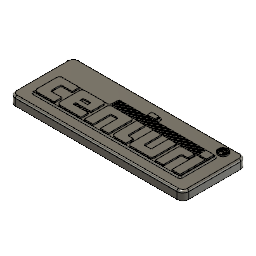
Centuri (Autodesk Fusion 360 design; units mm, degrees)
Autodesk Fusion 360 part; units mm, degrees
note: some values were not read from the file. Set by a fixed rule: which sketch regions a step uses.
sketch "Sketch1" plane through (0, 0, 0) normal (0, 1, 0) x (1, 0, 0)
  line L0 (168.1224, -0.1324) -> (6.1323, -0.1324)
  line L1 (0.1323, -6.1324) -> (0.1323, -58.135)
  line L2 (6.1323, -64.135) -> (168.1224, -64.135)
  line L3 (174.1224, -58.135) -> (174.1224, -6.1324)
  arc A0 (6.1323, -0.1324) -> (0.1323, -6.1324) centre (6.1323, -6.1324) ccw
  arc A1 (0.1323, -58.135) -> (6.1323, -64.135) centre (6.1323, -58.135) ccw
  arc A2 (174.1224, -6.1324) -> (168.1224, -0.1324) centre (168.1224, -6.1324) ccw
  arc A3 (168.1224, -64.135) -> (174.1224, -58.135) centre (168.1224, -58.135) ccw
  dimension "d26" = 6
  dimension "d27" = 6
  dimension "d28" = 6
  dimension "d29" = 6
  measures "d26" radius of A0
  measures "d27" radius of A1
  measures "d28" radius of A2
  measures "d29" radius of A3
extrude "Extrude1" add sketch "Sketch1" along normal blind 8.7
sketch "Sketch2" plane through (0, 8.7, 0) normal (0, 1, 0) x (-1, 0, 0)
  line L0 (-174.1224, 58.135) -> (-174.1224, 6.1324)
  line L1 (-168.1224, 0.1324) -> (-6.1323, 0.1324)
  line L2 (-0.1323, 6.1324) -> (-0.1323, 58.135)
  line L3 (-6.1323, 64.135) -> (-168.1224, 64.135)
  line L4 (-174.1224, 6.1324) -> (-174.1224, 58.135)
  line L5 (-168.1224, 64.135) -> (-6.1323, 64.135)
  line L6 (-0.1323, 58.135) -> (-0.1323, 6.1324)
  line L7 (-6.1323, 0.1324) -> (-168.1224, 0.1324)
  arc A0 (-168.1224, 64.135) -> (-174.1224, 58.135) centre (-168.1224, 58.135) ccw
  arc A1 (-174.1224, 6.1324) -> (-168.1224, 0.1324) centre (-168.1224, 6.1324) ccw
  arc A2 (-6.1323, 0.1324) -> (-0.1323, 6.1324) centre (-6.1323, 6.1324) ccw
  arc A3 (-0.1323, 58.135) -> (-6.1323, 64.135) centre (-6.1323, 58.135) ccw
  arc A4 (-168.1224, 64.135) -> (-174.1224, 58.135) centre (-168.1224, 58.135) ccw
  arc A5 (-0.1323, 58.135) -> (-6.1323, 64.135) centre (-6.1323, 58.135) ccw
  arc A6 (-6.1323, 0.1324) -> (-0.1323, 6.1324) centre (-6.1323, 6.1324) ccw
  arc A7 (-174.1224, 6.1324) -> (-168.1224, 0.1324) centre (-168.1224, 6.1324) ccw
  line L8 (-61.1568, 23.5465) -> (-61.1568, 18.1721)
  line L9 (-13.3787, 24.5465) -> (-60.1568, 24.5465)
  line L10 (-160.8508, 51.6795) -> (-160.8508, 18.1721)
  line L11 (-158.8508, 16.1721) -> (-101.0747, 16.1721)
  line L12 (-100.0747, 12.3992) -> (-100.0747, 15.1721)
  line L13 (-91.1387, 10.3992) -> (-98.0747, 10.3992)
  line L14 (-89.1387, 12.3992) -> (-89.1387, 15.1721)
  line L15 (-88.1387, 16.1721) -> (-63.1568, 16.1721)
  line L16 (-13.3787, 53.6795) -> (-158.8508, 53.6795)
  line L17 (-11.3787, 51.6795) -> (-11.3787, 26.5465)
  arc A8 (-63.1568, 16.1721) -> (-61.1568, 18.1721) centre (-63.1568, 18.1721) ccw
  arc A9 (-91.1387, 10.3992) -> (-89.1387, 12.3992) centre (-91.1387, 12.3992) ccw
  arc A10 (-100.0747, 12.3992) -> (-98.0747, 10.3992) centre (-98.0747, 12.3992) ccw
  arc A11 (-160.8508, 18.1721) -> (-158.8508, 16.1721) centre (-158.8508, 18.1721) ccw
  arc A12 (-158.8508, 53.6795) -> (-160.8508, 51.6795) centre (-158.8508, 51.6795) ccw
  arc A13 (-11.3787, 51.6795) -> (-13.3787, 53.6795) centre (-13.3787, 51.6795) ccw
  arc A14 (-13.3787, 24.5465) -> (-11.3787, 26.5465) centre (-13.3787, 26.5465) ccw
  arc A15 (-60.1568, 24.5465) -> (-61.1568, 23.5465) centre (-60.1568, 23.5465) ccw
  arc A16 (-88.1387, 16.1721) -> (-89.1387, 15.1721) centre (-88.1387, 15.1721) ccw
  arc A17 (-100.0747, 15.1721) -> (-101.0747, 16.1721) centre (-101.0747, 15.1721) ccw
  dimension "d32" = 2
  dimension "d33" = 2
  dimension "d34" = 2
  dimension "d35" = 2
  dimension "d36" = 2
  dimension "d37" = 2
  dimension "d38" = 2
  dimension "d39" = 1
  dimension "d40" = 1
  dimension "d41" = 1
  measures "d32" radius of A8
  measures "d33" radius of A9
  measures "d34" radius of A10
  measures "d35" radius of A11
  measures "d36" radius of A12
  measures "d37" radius of A13
  measures "d38" radius of A14
  measures "d39" radius of A15
  measures "d40" radius of A16
  measures "d41" radius of A17
extrude "Extrude2" add sketch "Sketch2" along normal blind 1.2 contours L8 L9 L10 L11 L12 L13 L14 L15 L16 L17 A8 A9 A10 A11 A12 A13 A14 A15 A16 A17
sketch "Sketch3" plane through (0, 9.9, 0) normal (0, 1, 0) x (-1, 0, 0)
  spline S0 degree 2 poles (-32.9928, 26.8178) (-19.083, 26.7952) (-15.8247, 26.8178) knots 0 0 0 1 1 1
  spline S1 degree 3 poles (-15.8247, 26.8178) (-14.6011, 26.8261) (-13.0709, 27.9977) (-13.0639, 29.2054) knots 0 0 0 0 1 1 1 1
  spline S2 degree 3 poles (-13.0639, 29.2054) (-13.0417, 32.9886) (-13.0526, 45.265) (-13.0639, 49.042) knots 0 0 0 0 1 1 1 1
  spline S3 degree 3 poles (-13.0639, 49.042) (-13.0677, 50.37) (-14.4791, 51.9469) (-15.8247, 51.9487) knots 0 0 0 0 1 1 1 1
  spline S4 degree 2 poles (-15.8247, 51.9487) (-19.0795, 51.9532) (-32.9674, 51.9487) knots 0 0 0 1 1 1
  line L0 (-32.9674, 51.9487) -> (-32.9928, 44.3788)
  spline S5 degree 2 poles (-32.9928, 44.3788) (-24.5516, 44.3725) (-22.6517, 44.3788) knots 0 0 0 1 1 1
  spline S6 degree 3 poles (-22.6517, 44.3788) (-22.0091, 44.3809) (-21.5788, 43.4319) (-21.5873, 42.7928) knots 0 0 0 0 1 1 1 1
  spline S7 degree 3 poles (-21.5873, 42.7928) (-21.6066, 41.3105) (-21.5967, 36.9365) (-21.5873, 35.4147) knots 0 0 0 0 1 1 1 1
  spline S8 degree 3 poles (-21.5873, 35.4147) (-21.5834, 34.8089) (-22.0316, 33.8745) (-22.6453, 33.8752) knots 0 0 0 0 1 1 1 1
  spline S9 degree 2 poles (-22.6453, 33.8752) (-24.5882, 33.8783) (-32.9928, 33.8752) knots 0 0 0 1 1 1
  line L1 (-32.9928, 33.8752) -> (-32.9928, 26.8178)
  spline S10 degree 3 poles (-56.7768, 26.8178) (-53.3593, 26.806) (-42.7162, 26.8025) (-39.2193, 26.8178) knots 0 0 0 0 1 1 1 1
  spline S11 degree 3 poles (-39.2193, 26.8178) (-37.8445, 26.8237) (-35.8622, 27.8316) (-35.8661, 29.1884) knots 0 0 0 0 1 1 1 1
  spline S12 degree 3 poles (-35.8661, 29.1884) (-35.8777, 33.0541) (-35.8672, 45.7175) (-35.8661, 49.4432) knots 0 0 0 0 1 1 1 1
  spline S13 degree 3 poles (-35.8661, 49.4432) (-35.8658, 50.8266) (-37.8171, 51.9476) (-39.2193, 51.9487) knots 0 0 0 0 1 1 1 1
  spline S14 degree 2 poles (-39.2193, 51.9487) (-43.0994, 51.9508) (-59.7334, 51.9487) knots 0 0 0 1 1 1
  line L2 (-59.7334, 51.9487) -> (-59.7334, 44.3788)
  spline S15 degree 2 poles (-59.7334, 44.3788) (-47.3321, 44.3802) (-44.8507, 44.3788) knots 0 0 0 1 1 1
  spline S16 degree 3 poles (-44.8507, 44.3788) (-44.0281, 44.3781) (-44.0281, 41.943) (-44.8507, 41.944) knots 0 0 0 0 1 1 1 1
  spline S17 degree 2 poles (-44.8507, 41.944) (-47.3567, 41.9471) (-59.7334, 41.944) knots 0 0 0 1 1 1
  spline S18 degree 2 poles (-59.7334, 41.944) (-59.732, 31.8277) (-59.7334, 29.1884) knots 0 0 0 1 1 1
  spline S19 degree 3 poles (-59.7334, 29.1884) (-59.7342, 27.9349) (-58.0465, 26.8219) (-56.7768, 26.8178) knots 0 0 0 0 1 1 1 1
  line L3 (-44.6029, 37.6033) -> (-52.1177, 37.6033)
  spline S20 degree 2 poles (-52.1177, 37.6033) (-52.1195, 35.5658) (-52.1177, 35.0104) knots 0 0 0 1 1 1
  spline S21 degree 3 poles (-52.1177, 35.0104) (-52.117, 34.6915) (-51.7641, 34.3481) (-51.4621, 34.3488) knots 0 0 0 0 1 1 1 1
  spline S22 degree 3 poles (-51.4621, 34.3488) (-50.3271, 34.3526) (-46.4378, 34.3473) (-45.2915, 34.3488) knots 0 0 0 0 1 1 1 1
  spline S23 degree 3 poles (-45.2915, 34.3488) (-44.9814, 34.3496) (-44.6039, 34.683) (-44.6029, 35.0104) knots 0 0 0 0 1 1 1 1
  spline S24 degree 2 poles (-44.6029, 35.0104) (-44.6011, 35.5814) (-44.6029, 37.6033) knots 0 0 0 1 1 1
  line L4 (-63.1696, 51.9483) -> (-71.8638, 51.9483)
  spline S25 degree 2 poles (-71.8638, 51.9483) (-71.8656, 38.5103) (-71.8638, 35.6595) knots 0 0 0 1 1 1
  spline S26 degree 3 poles (-71.8638, 35.6595) (-71.8634, 34.7649) (-71.8395, 34.1505) (-72.4016, 34.1501) knots 0 0 0 0 1 1 1 1
  spline S27 degree 3 poles (-72.4016, 34.1501) (-73.5093, 34.1491) (-77.3834, 34.1456) (-78.5466, 34.1501) knots 0 0 0 0 1 1 1 1
  spline S28 degree 3 poles (-78.5466, 34.1501) (-79.1909, 34.1526) (-79.1888, 34.8162) (-79.1895, 35.6595) knots 0 0 0 0 1 1 1 1
  spline S29 degree 2 poles (-79.1895, 35.6595) (-79.1923, 38.6438) (-79.1895, 51.9071) knots 0 0 0 1 1 1
  line L5 (-79.1895, 51.9071) -> (-87.5653, 51.9483)
  spline S30 degree 2 poles (-87.5653, 51.9483) (-87.5688, 33.4546) (-87.5653, 29.1884) knots 0 0 0 1 1 1
  spline S31 degree 3 poles (-87.5653, 29.1884) (-87.5646, 28.1107) (-86.4298, 26.8171) (-85.3377, 26.8178) knots 0 0 0 0 1 1 1 1
  spline S32 degree 3 poles (-85.3377, 26.8178) (-81.607, 26.8202) (-69.4534, 26.8101) (-65.7431, 26.8178) knots 0 0 0 0 1 1 1 1
  spline S33 degree 3 poles (-65.7431, 26.8178) (-64.5697, 26.8202) (-63.1696, 28.0306) (-63.1696, 29.1884) knots 0 0 0 0 1 1 1 1
  spline S34 degree 2 poles (-63.1696, 29.1884) (-63.1689, 33.4147) (-63.1696, 51.9483) knots 0 0 0 1 1 1
  line L6 (-90.6576, 26.8178) -> (-98.9156, 26.8178)
  spline S35 degree 2 poles (-98.9156, 26.8178) (-98.9159, 40.6126) (-98.9156, 43.5182) knots 0 0 0 1 1 1
  spline S36 degree 3 poles (-98.9156, 43.5182) (-98.9152, 43.9294) (-99.3947, 44.3788) (-99.8116, 44.3788) knots 0 0 0 0 1 1 1 1
  spline S37 degree 2 poles (-99.8116, 44.3788) (-99.8559, 44.3788) (-104.8904, 44.3788) knots 0 0 0 1 1 1
  line L7 (-104.8904, 44.3788) -> (-104.946, 51.9532)
  spline S38 degree 2 poles (-104.946, 51.9532) (-96.959, 51.9452) (-94.523, 51.9532) knots 0 0 0 1 1 1
  spline S39 degree 3 poles (-94.523, 51.9532) (-90.2713, 51.9667) (-90.6439, 48.9779) (-90.6435, 47.4106) knots 0 0 0 0 1 1 1 1
  spline S40 degree 2 poles (-90.6435, 47.4106) (-90.6425, 43.2176) (-90.6576, 26.8178) knots 0 0 0 1 1 1
  line L8 (-107.072, 26.8178) -> (-115.2878, 26.8178)
  spline S41 degree 2 poles (-115.2878, 26.8178) (-115.2881, 40.5276) (-115.2878, 43.4547) knots 0 0 0 1 1 1
  spline S42 degree 3 poles (-115.2878, 43.4547) (-115.2878, 43.8323) (-115.5693, 44.3784) (-115.9521, 44.3788) knots 0 0 0 0 1 1 1 1
  spline S43 degree 3 poles (-115.9521, 44.3788) (-117.0559, 44.3791) (-120.8583, 44.3788) (-121.979, 44.3788) knots 0 0 0 0 1 1 1 1
  spline S44 degree 3 poles (-121.979, 44.3788) (-122.3375, 44.3788) (-122.508, 43.8084) (-122.5084, 43.4547) knots 0 0 0 0 1 1 1 1
  spline S45 degree 2 poles (-122.5084, 43.4547) (-122.5105, 40.5287) (-122.5084, 26.8178) knots 0 0 0 1 1 1
  line L9 (-122.5084, 26.8178) -> (-130.83, 26.8178)
  spline S46 degree 2 poles (-130.83, 26.8178) (-130.8286, 44.9394) (-130.83, 49.1325) knots 0 0 0 1 1 1
  spline S47 degree 3 poles (-130.83, 49.1325) (-130.8303, 50.3291) (-129.8661, 51.9483) (-128.543, 51.9494) knots 0 0 0 0 1 1 1 1
  spline S48 degree 3 poles (-128.543, 51.9494) (-124.6333, 51.9528) (-112.8693, 51.9521) (-109.3164, 51.9494) knots 0 0 0 0 1 1 1 1
  spline S49 degree 3 poles (-109.3164, 51.9494) (-108.0865, 51.9487) (-107.0706, 50.2577) (-107.072, 49.1328) knots 0 0 0 0 1 1 1 1
  spline S50 degree 2 poles (-107.072, 49.1328) (-107.0765, 44.9318) (-107.072, 26.8178) knots 0 0 0 1 1 1
  line L10 (-148.6286, 26.8178) -> (-148.6286, 33.5954)
  spline S51 degree 2 poles (-148.6286, 33.5954) (-144.7896, 33.5968) (-143.7112, 33.5954) knots 0 0 0 1 1 1
  spline S52 degree 3 poles (-143.7112, 33.5954) (-142.9807, 33.5943) (-142.2763, 34.5093) (-142.2756, 35.2306) knots 0 0 0 0 1 1 1 1
  spline S53 degree 2 poles (-142.2756, 35.2306) (-142.2735, 38.3037) (-142.2756, 51.9521) knots 0 0 0 1 1 1
  line L11 (-142.2756, 51.9521) -> (-134.2615, 51.9521)
  spline S54 degree 2 poles (-134.2615, 51.9521) (-134.2622, 33.6976) (-134.2615, 29.4065) knots 0 0 0 1 1 1
  spline S55 degree 3 poles (-134.2615, 29.4065) (-134.2612, 27.9849) (-136.2557, 26.8198) (-137.6963, 26.8178) knots 0 0 0 0 1 1 1 1
  spline S56 degree 2 poles (-137.6963, 26.8178) (-140.0743, 26.8143) (-148.6286, 26.8178) knots 0 0 0 1 1 1
  line L12 (-150.7694, 26.8178) -> (-159.0611, 26.8178)
  line L13 (-159.0611, 26.8178) -> (-159.0611, 51.949)
  line L14 (-159.0611, 51.949) -> (-150.7694, 51.8679)
  line L15 (-150.7694, 51.8679) -> (-150.7694, 26.8178)
  spline S57 degree 3 poles (-98.4051, 12.6404) (-98.4051, 12.3033) (-98.1313, 12.0297) (-97.7942, 12.0297) knots 0 0 0 0 1 1 1 1
  line L16 (-97.7942, 12.0297) -> (-91.45, 12.0297)
  spline S58 degree 3 poles (-91.45, 12.0297) (-91.113, 12.0297) (-90.8394, 12.3033) (-90.8394, 12.6404) knots 0 0 0 0 1 1 1 1
  line L17 (-90.8394, 12.6404) -> (-90.8394, 15.7818)
  spline S59 degree 3 poles (-90.8394, 15.7818) (-90.8394, 16.1189) (-91.113, 16.3927) (-91.45, 16.3927) knots 0 0 0 0 1 1 1 1
  line L18 (-91.45, 16.3927) -> (-97.7942, 16.3927)
  spline S60 degree 3 poles (-97.7942, 16.3927) (-98.1313, 16.3927) (-98.4051, 16.1189) (-98.4051, 15.7818) knots 0 0 0 0 1 1 1 1
  line L19 (-98.4051, 15.7818) -> (-98.4051, 12.6404)
  spline S61 degree 2 poles (-64.6658, 17.7949) (-80.3905, 17.7962) (-159.0863, 17.7949) knots 0 0 0 1 1 1
  line L20 (-159.0863, 17.7949) -> (-159.0863, 25.3701)
  spline S62 degree 2 poles (-159.0863, 25.3701) (-80.3944, 25.3701) (-64.6658, 25.3701) knots 0 0 0 1 1 1
  spline S63 degree 3 poles (-64.6658, 25.3701) (-64.173, 25.3701) (-64.1386, 24.2219) (-64.6658, 24.2219) knots 0 0 0 0 1 1 1 1
  spline S64 degree 3 poles (-64.6658, 24.2219) (-79.0329, 24.2233) (-136.3969, 24.2233) (-150.7538, 24.2219) knots 0 0 0 0 1 1 1 1
  spline S65 degree 3 poles (-150.7538, 24.2219) (-151.4642, 24.2219) (-151.4593, 23.1496) (-150.7538, 23.153) knots 0 0 0 0 1 1 1 1
  spline S66 degree 3 poles (-150.7538, 23.153) (-136.4039, 23.2243) (-78.9781, 23.1647) (-64.6658, 23.153) knots 0 0 0 0 1 1 1 1
  spline S67 degree 3 poles (-64.6658, 23.153) (-64.1649, 23.1526) (-64.1765, 22.084) (-64.6658, 22.084) knots 0 0 0 0 1 1 1 1
  spline S68 degree 3 poles (-64.6658, 22.084) (-79.0139, 22.0837) (-136.3853, 22.0789) (-150.7538, 22.084) knots 0 0 0 0 1 1 1 1
  spline S69 degree 3 poles (-150.7538, 22.084) (-151.4976, 22.084) (-151.4603, 21.0151) (-150.7538, 21.0151) knots 0 0 0 0 1 1 1 1
  spline S70 degree 3 poles (-150.7538, 21.0151) (-136.3853, 21.0141) (-78.9971, 21.0158) (-64.6658, 21.0151) knots 0 0 0 0 1 1 1 1
  spline S71 degree 3 poles (-64.6658, 21.0151) (-64.1589, 21.0148) (-64.1916, 19.9461) (-64.6658, 19.9458) knots 0 0 0 0 1 1 1 1
  spline S72 degree 3 poles (-64.6658, 19.9458) (-79.022, 19.94) (-136.3582, 19.9468) (-150.7538, 19.9458) knots 0 0 0 0 1 1 1 1
  spline S73 degree 3 poles (-150.7538, 19.9458) (-151.4023, 19.9458) (-151.4044, 18.8769) (-150.7538, 18.8769) knots 0 0 0 0 1 1 1 1
  spline S74 degree 3 poles (-150.7538, 18.8769) (-136.4039, 18.8796) (-79.0333, 18.8727) (-64.6658, 18.8769) knots 0 0 0 0 1 1 1 1
  spline S75 degree 3 poles (-64.6658, 18.8769) (-64.1625, 18.8772) (-64.167, 17.7945) (-64.6658, 17.7949) knots 0 0 0 0 1 1 1 1
  line L21 (-61.1568, 18.1721) -> (-61.1568, 23.5465)
  line L22 (-60.1568, 24.5465) -> (-13.3787, 24.5465)
  arc A0 (-100.0747, 12.3992) -> (-98.0747, 10.3992) centre (-98.0747, 12.3992) ccw
  line L23 (-98.0747, 10.3992) -> (-91.1387, 10.3992)
  arc A1 (-91.1387, 10.3992) -> (-89.1387, 12.3992) centre (-91.1387, 12.3992) ccw
  line L24 (-89.1387, 12.3992) -> (-89.1387, 15.1721)
  arc A2 (-88.1387, 16.1721) -> (-89.1387, 15.1721) centre (-88.1387, 15.1721) ccw
  line L25 (-88.1387, 16.1721) -> (-63.1568, 16.1721)
  arc A3 (-63.1568, 16.1721) -> (-61.1568, 18.1721) centre (-63.1568, 18.1721) ccw
  arc A4 (-60.1568, 24.5465) -> (-61.1568, 23.5465) centre (-60.1568, 23.5465) ccw
  arc A5 (-13.3787, 24.5465) -> (-11.3787, 26.5465) centre (-13.3787, 26.5465) ccw
  line L26 (-11.3787, 26.5465) -> (-11.3787, 51.6795)
  arc A6 (-11.3787, 51.6795) -> (-13.3787, 53.6795) centre (-13.3787, 51.6795) ccw
  line L27 (-13.3787, 53.6795) -> (-158.8508, 53.6795)
  arc A7 (-158.8508, 53.6795) -> (-160.8508, 51.6795) centre (-158.8508, 51.6795) ccw
  line L28 (-160.8508, 51.6795) -> (-160.8508, 18.1721)
  arc A8 (-160.8508, 18.1721) -> (-158.8508, 16.1721) centre (-158.8508, 18.1721) ccw
  line L29 (-158.8508, 16.1721) -> (-101.0747, 16.1721)
  arc A9 (-100.0747, 15.1721) -> (-101.0747, 16.1721) centre (-101.0747, 15.1721) ccw
  line L30 (-100.0747, 15.1721) -> (-100.0747, 12.3992)
extrude "Extrude3" add sketch "Sketch3" along normal blind 1.25 contours S0 S1 S2 S3 S4 L0 S5 S6 S7 S8 S9 L1 | S10 S11 S12 S13 S14 L2 S15 S16 S17 S18 S19 | L4 S25 S26 S27 S28 S29 L5 S30 S31 S32 S33 S34 | L6 S35 S36 S37 L7 S38 S39 S40 | L8 S41 S42 S43 S44 S45 L9 S46 S47 S48 S49 S50 | L10 S51 S52 S53 L11 S54 S55 S56 | L12 L13 L14 L15 | S57 L16 S58 L17 S59 L18 S60 L19 | S61 L20 S62 S63 S64 S65 S66 S67 S68 S69 S70 S71 S72 S73 S74 S75
sketch "Sketch4" plane through (0, 8.7, 0) normal (0, 1, 0) x (-1, 0, 0)
  circle A0 centre (-159.5007, 9.1533) radius 4.7474
  arc A1 (-6.1323, 0.1324) -> (-0.1323, 6.1324) centre (-6.1323, 6.1324) ccw
  arc A2 (-0.1323, 58.135) -> (-6.1323, 64.135) centre (-6.1323, 58.135) ccw
  arc A3 (-168.1224, 64.135) -> (-174.1224, 58.135) centre (-168.1224, 58.135) ccw
  arc A4 (-174.1224, 6.1324) -> (-168.1224, 0.1324) centre (-168.1224, 6.1324) ccw
  line L0 (-61.1568, 23.5465) -> (-61.1568, 18.1721)
  line L1 (-13.3787, 24.5465) -> (-60.1568, 24.5465)
  line L2 (-174.1224, 58.135) -> (-174.1224, 6.1324)
  line L3 (-168.1224, 0.1324) -> (-6.1323, 0.1324)
  line L4 (-0.1323, 6.1324) -> (-0.1323, 58.135)
  line L5 (-6.1323, 64.135) -> (-168.1224, 64.135)
  line L6 (-100.0747, 12.3992) -> (-100.0747, 15.1721)
  arc A5 (-100.0747, 15.1721) -> (-101.0747, 16.1721) centre (-101.0747, 15.1721) ccw
  line L7 (-101.0747, 16.1721) -> (-158.8508, 16.1721)
  arc A6 (-160.8508, 18.1721) -> (-158.8508, 16.1721) centre (-158.8508, 18.1721) ccw
  line L8 (-160.8508, 18.1721) -> (-160.8508, 51.6795)
  arc A7 (-158.8508, 53.6795) -> (-160.8508, 51.6795) centre (-158.8508, 51.6795) ccw
  line L9 (-158.8508, 53.6795) -> (-13.3787, 53.6795)
  arc A8 (-11.3787, 51.6795) -> (-13.3787, 53.6795) centre (-13.3787, 51.6795) ccw
  line L10 (-11.3787, 51.6795) -> (-11.3787, 26.5465)
  arc A9 (-13.3787, 24.5465) -> (-11.3787, 26.5465) centre (-13.3787, 26.5465) ccw
  arc A10 (-60.1568, 24.5465) -> (-61.1568, 23.5465) centre (-60.1568, 23.5465) ccw
  arc A11 (-63.1568, 16.1721) -> (-61.1568, 18.1721) centre (-63.1568, 18.1721) ccw
  line L11 (-63.1568, 16.1721) -> (-88.1387, 16.1721)
  arc A12 (-88.1387, 16.1721) -> (-89.1387, 15.1721) centre (-88.1387, 15.1721) ccw
  line L12 (-89.1387, 15.1721) -> (-89.1387, 12.3992)
  arc A13 (-91.1387, 10.3992) -> (-89.1387, 12.3992) centre (-91.1387, 12.3992) ccw
  line L13 (-91.1387, 10.3992) -> (-98.0747, 10.3992)
  arc A14 (-100.0747, 12.3992) -> (-98.0747, 10.3992) centre (-98.0747, 12.3992) ccw
extrude "Extrude4" add sketch "Sketch4" along normal blind 1.25 contours A0
sketch "Sketch5" plane through (0, 9.95, 0) normal (0, 1, 0) x (-1, 0, 0)
  circle A0 centre (-159.5007, 9.1533) radius 4.7474
  circle A1 centre (-159.5007, 9.1533) radius 3.625
  dimension "d11" = 7.25
  measures "d11" diameter of A1
sketch "Sketch6" plane through (0, 9.95, 0) normal (0, 1, 0) x (-1, 0, 0)
  circle A0 centre (-159.5007, 9.1533) radius 4.7474
  circle A1 centre (-159.5007, 9.1533) radius 4
  dimension "d14" = 8
  measures "d14" diameter of A1
extrude "Extrude6" cut sketch "Sketch6" against normal blind 0.5 contours A1
sketch "Sketch10" plane through (0, 8.7, 0) normal (0, 1, 0) x (-1, 0, 0)
  circle A0 centre (-159.5007, 9.1533) radius 4.7474
  line L0 (-157.9472, 11.8222) -> (-157.2705, 11.8241)
  line L1 (-157.2705, 11.8241) -> (-157.2792, 6.5593)
  line L2 (-157.2792, 6.5593) -> (-161.0179, 6.552)
  spline S0 degree 2 poles (-161.0179, 6.552) (-161.3183, 6.552) (-161.4788, 6.5509) knots 0 0 0 1 1 1
  spline S1 degree 3 poles (-161.4788, 6.5509) (-161.764, 6.549) (-162.319, 7.2818) (-162.3366, 8.0212) knots 0 0 0 0 1 1 1 1
  spline S2 degree 3 poles (-162.3366, 8.0212) (-162.3591, 8.9834) (-161.7629, 9.6698) (-161.4674, 9.6733) knots 0 0 0 0 1 1 1 1
  spline S3 degree 2 poles (-161.4674, 9.6733) (-161.2646, 9.6758) (-161.006, 9.6687) knots 0 0 0 1 1 1
  line L3 (-161.006, 9.6687) -> (-161.9004, 11.8106)
  line L4 (-161.9004, 11.8106) -> (-161.2174, 11.8106)
  line L5 (-161.2174, 11.8106) -> (-160.3415, 9.6687)
  line L6 (-160.3415, 9.6687) -> (-157.9416, 9.6644)
  line L7 (-157.9416, 9.6644) -> (-157.9472, 11.8222)
  line L8 (-157.9518, 7.1869) -> (-160.8281, 7.1728)
  spline S4 degree 2 poles (-160.8281, 7.1728) (-160.9225, 7.1709) (-160.9637, 7.172) knots 0 0 0 1 1 1
  spline S5 degree 3 poles (-160.9637, 7.172) (-161.1212, 7.1761) (-161.6233, 7.3664) (-161.6228, 8.0174) knots 0 0 0 0 1 1 1 1
  spline S6 degree 3 poles (-161.6228, 8.0174) (-161.622, 8.9253) (-161.1326, 8.9573) (-160.9637, 8.9592) knots 0 0 0 0 1 1 1 1
  spline S7 degree 2 poles (-160.9637, 8.9592) (-160.8851, 8.96) (-160.8222, 8.9584) knots 0 0 0 1 1 1
  line L9 (-160.8222, 8.9584) -> (-157.9543, 8.944)
  line L10 (-157.9543, 8.944) -> (-157.9518, 7.1869)
  arc A1 (-6.1323, 0.1324) -> (-0.1323, 6.1324) centre (-6.1323, 6.1324) ccw
  arc A2 (-0.1323, 58.135) -> (-6.1323, 64.135) centre (-6.1323, 58.135) ccw
  arc A3 (-168.1224, 64.135) -> (-174.1224, 58.135) centre (-168.1224, 58.135) ccw
  arc A4 (-174.1224, 6.1324) -> (-168.1224, 0.1324) centre (-168.1224, 6.1324) ccw
  line L11 (-61.1568, 23.5465) -> (-61.1568, 18.1721)
  line L12 (-13.3787, 24.5465) -> (-60.1568, 24.5465)
  line L13 (-174.1224, 58.135) -> (-174.1224, 6.1324)
  line L14 (-168.1224, 0.1324) -> (-6.1323, 0.1324)
  line L15 (-0.1323, 6.1324) -> (-0.1323, 58.135)
  line L16 (-6.1323, 64.135) -> (-168.1224, 64.135)
  line L17 (-100.0747, 12.3992) -> (-100.0747, 15.1721)
  arc A5 (-100.0747, 15.1721) -> (-101.0747, 16.1721) centre (-101.0747, 15.1721) ccw
  line L18 (-101.0747, 16.1721) -> (-158.8508, 16.1721)
  arc A6 (-160.8508, 18.1721) -> (-158.8508, 16.1721) centre (-158.8508, 18.1721) ccw
  line L19 (-160.8508, 18.1721) -> (-160.8508, 51.6795)
  arc A7 (-158.8508, 53.6795) -> (-160.8508, 51.6795) centre (-158.8508, 51.6795) ccw
  line L20 (-158.8508, 53.6795) -> (-13.3787, 53.6795)
  arc A8 (-11.3787, 51.6795) -> (-13.3787, 53.6795) centre (-13.3787, 51.6795) ccw
  line L21 (-11.3787, 51.6795) -> (-11.3787, 26.5465)
  arc A9 (-13.3787, 24.5465) -> (-11.3787, 26.5465) centre (-13.3787, 26.5465) ccw
  arc A10 (-60.1568, 24.5465) -> (-61.1568, 23.5465) centre (-60.1568, 23.5465) ccw
  arc A11 (-63.1568, 16.1721) -> (-61.1568, 18.1721) centre (-63.1568, 18.1721) ccw
  line L22 (-63.1568, 16.1721) -> (-88.1387, 16.1721)
  arc A12 (-88.1387, 16.1721) -> (-89.1387, 15.1721) centre (-88.1387, 15.1721) ccw
  line L23 (-89.1387, 15.1721) -> (-89.1387, 12.3992)
  arc A13 (-91.1387, 10.3992) -> (-89.1387, 12.3992) centre (-91.1387, 12.3992) ccw
  line L24 (-91.1387, 10.3992) -> (-98.0747, 10.3992)
  arc A14 (-100.0747, 12.3992) -> (-98.0747, 10.3992) centre (-98.0747, 12.3992) ccw
extrude "Extrude9" add sketch "Sketch10" along normal blind 1.25 contours L0 L1 L2 S0 S1 S2 S3 L3 L4 L5 L6 L7
fillet "Fillet4" radius 1.8 8 edges at (172.365, 8.7, 1.8897) (87.1273, 8.7, 0.1324) (1.8896, 8.7, 1.8897) (0.1323, 8.7, 32.1337) (1.8896, 8.7, 62.3777) (87.1273, 8.7, 64.135) (172.365, 8.7, 62.3777) (174.1224, 8.7, 32.1337)
fillet "Fillet5" radius 1.2 20 edges at (160.8508, 9.9, 34.9258) (160.265, 9.9, 16.7579) (129.9627, 9.9, 16.1721) (100.3676, 9.9, 15.8792) (100.0747, 9.9, 13.7857) (99.4889, 9.9, 10.985) (94.6067, 9.9, 10.3992) (89.7244, 9.9, 10.985) (89.1387, 9.9, 13.7857) (88.8458, 9.9, 15.8792) (75.6477, 9.9, 16.1721) (61.7425, 9.9, 16.7579) (61.1568, 9.9, 20.8593) (60.8639, 9.9, 24.2536) (36.7677, 9.9, 24.5465) (11.9645, 9.9, 25.1322) (11.3787, 9.9, 39.113) (11.9645, 9.9, 53.0937) (86.1148, 9.9, 53.6795) (160.265, 9.9, 53.0937)
